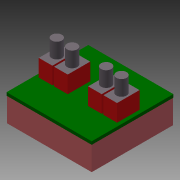
# Autodesk Inventor part: ccpdu
Saved by Autodesk Inventor 2013 SP2 (Build 170200200, 200)
## iProperties
Created: 2019-01-29
Part Number: ccpdu
Material: Generic
Document SubType Name: Modeling
Designer: alex
Density: 1 g/cm^3
Author: alex
Autodesk Inventor part; units mm, degrees
ref_plane "YZ Plane" through (0, 0, 0) normal (1, 0, 0) x (0, 1, 0)
ref_plane "XZ Plane" through (0, 0, 0) normal (0, 1, 0) x (-1, 0, 0)
ref_plane "XY Plane" through (0, 0, 0) normal (0, 0, 1) x (1, 0, 0)
sketch "Sketch1" plane through (0, 0, 0) normal (0, 1, 0) x (-1, 0, 0)
  line L0 (0, 0) -> (50, 0)
  line L1 (50, 0) -> (50, 48)
  line L2 (50, 48) -> (0, 48)
  line L3 (0, 48) -> (0, 0)
  dimension "d0" = 50
  dimension "d1" = 48
  constraints: 8 end point, 2 parallel, 1 horizontal, 1 perpendicular
  measures "d0" distance of L0.start L0.end
  measures "d1" distance of L2.end L0.start
extrude "Extrusion1" add sketch "Sketch1" along normal blind 1.8
sketch "Sketch4" plane through (0, 1.8, 0) normal (0, 1, 0) x (1, 0, 0)
  line L0 (0, 0) -> (-50, 0) projected
  line L1 (-50, 0) -> (-50, -48) projected
  line L2 (-48, -17.9) -> (-40, -17.9)
  line L3 (-40, -17.9) -> (-40, -31.1)
  line L4 (-40, -31.1) -> (-48, -31.1)
  line L5 (-48, -31.1) -> (-48, -17.9)
  line L6 (-44, -24.5) -> (-44, -17.9)
  line L7 (-44, -24.5) -> (-40, -24.5)
  line L8 (-44, -24.5) -> (-44, -31.1)
  line L9 (-44, -24.5) -> (-48, -24.5)
  line L10 (-39, -17.9) -> (-31, -17.9)
  line L11 (-31, -17.9) -> (-31, -31.1)
  line L12 (-31, -31.1) -> (-39, -31.1)
  line L13 (-39, -31.1) -> (-39, -17.9)
  line L14 (-35, -24.5) -> (-35, -17.9)
  line L15 (-35, -24.5) -> (-31, -24.5)
  line L16 (-35, -24.5) -> (-35, -31.1)
  line L17 (-35, -24.5) -> (-39, -24.5)
  line L18 (-19, -17.9) -> (-11, -17.9)
  line L19 (-11, -17.9) -> (-11, -31.1)
  line L20 (-11, -31.1) -> (-19, -31.1)
  line L21 (-19, -31.1) -> (-19, -17.9)
  line L22 (-15, -24.5) -> (-15, -17.9)
  line L23 (-15, -24.5) -> (-11, -24.5)
  line L24 (-15, -24.5) -> (-15, -31.1)
  line L25 (-15, -24.5) -> (-19, -24.5)
  line L26 (-2, -17.9) -> (-2, -31.1)
  line L27 (-6, -24.5) -> (-6, -17.9)
  line L28 (-6, -24.5) -> (-2, -24.5)
  line L29 (-6, -24.5) -> (-6, -31.1)
  line L30 (-2, -31.1) -> (-10, -31.1)
  line L31 (-10, -17.9) -> (-2, -17.9)
  line L32 (-6, -24.5) -> (-10, -24.5)
  line L33 (-10, -31.1) -> (-10, -17.9)
  dimension "d4" = 8
  dimension "d6" = 13.2
  dimension "d7" = 24.5
  dimension "d8" = 6
  dimension "d9" = 8
  dimension "d10" = 13.2
  dimension "d12" = 9
  dimension "d13" = 8
  dimension "d14" = 13.2
  dimension "d15" = 8
  dimension "d16" = 13.2
  dimension "d17" = 20
  dimension "d18" = 9
  constraints: 64 end point, 20 perpendicular, 16 midpoint, 8 collinear, 8 parallel, 4 horizontal
  measures "d4" distance of L3.end L4.end
  measures "d6" distance of L2.end L3.end
  measures "d7" distance from line of L0 L6.start
  measures "d8" distance from line of L1 L6.start
  measures "d9" distance of L11.end L12.end
  measures "d10" distance of L10.end L11.end
  measures "d12" distance of L14.start L6.start
  measures "d13" distance of L19.end L20.end
  measures "d14" distance of L19.start L19.end
  measures "d15" distance of L30.start L33.start
  measures "d16" distance of L26.start L30.start
  measures "d17" distance from line of L14 L22.start
  measures "d18" distance of L22.start L29.start
extrude "Extrusion2" add sketch "Sketch4" along normal blind 10
sketch "Sketch5" plane through (0, 11.8, 0) normal (0, 1, 0) x (1, 0, 0)
  line L0 (-31, -31.1) -> (-31, -17.9) projected
  line L1 (-31, -17.9) -> (-39, -17.9) projected
  line L2 (-39, -17.9) -> (-39, -31.1) projected
  line L3 (-39, -31.1) -> (-31, -31.1) projected
  line L4 (-11, -31.1) -> (-11, -17.9) projected
  line L5 (-11, -17.9) -> (-19, -17.9) projected
  line L6 (-19, -17.9) -> (-19, -31.1) projected
  line L7 (-19, -31.1) -> (-11, -31.1) projected
  line L8 (-2, -17.9) -> (-10, -17.9) projected
  line L9 (-10, -17.9) -> (-10, -31.1) projected
  line L10 (-10, -31.1) -> (-2, -31.1) projected
  line L11 (-2, -31.1) -> (-2, -17.9) projected
  circle A0 centre (-44, -24.5) radius 3
  circle A1 centre (-35, -24.5) radius 3
  circle A2 centre (-15, -24.5) radius 3
  circle A3 centre (-6, -24.5) radius 3
  point P0 (0, 0)
  dimension "d21" = 6
  dimension "d23" = 6
  dimension "d24" = 6
  dimension "d25" = 6
  constraints: 4 centre point
  measures "d21" diameter of A0
  measures "d23" diameter of A1
  measures "d24" diameter of A2
  measures "d25" diameter of A3
extrude "Extrusion3" add sketch "Sketch5" along normal blind 9 contours A0 | A1 | A2 | A3
sketch "Sketch6" plane through (0, 0, 0) normal (0, -1, 0) x (1, 0, 0)
  line L0 (0, 0) -> (-50, 0) projected
  line L1 (0, 48) -> (0, 0) projected
  line L2 (-50, 48) -> (0, 48) projected
  line L3 (-50, 0) -> (-50, 48) projected
  line L4 (-0.1, 47.9) -> (-0.1, 0.1)
  line L5 (-0.1, 0.1) -> (-49.9, 0.1)
  line L6 (-49.9, 0.1) -> (-49.9, 47.9)
  line L7 (-49.9, 47.9) -> (-0.1, 47.9)
  dimension "d28" = 0.1
  constraints: 8 end point, 3 other
  measures "d28" distance between parallel lines of L2 L7
extrude "Extrusion4" add sketch "Sketch6" along normal blind 14 contours L4 L5 L6 L7
body "Solid1"
